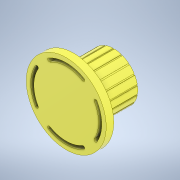
# Autodesk Inventor part: 3inPvcCap
Saved by Autodesk Inventor 2022.2 (Build 262287000, 287)
## iProperties
Created: 2021-11-22
Part Number: 3inPvcCap
Material: PC/ABS Plastic
Document SubType Name: Modeling
Designer: robst
Density: 0.357273 g/cm^3
Appearance: Smooth - Yellow
Author: robst
Autodesk Inventor part; units mm, degrees
ref_plane "YZ Plane" through (0, 0, 0) normal (1, 0, 0) x (0, 1, 0)
ref_plane "XZ Plane" through (0, 0, 0) normal (0, 1, 0) x (-1, 0, 0)
ref_plane "XY Plane" through (0, 0, 0) normal (0, 0, 1) x (1, 0, 0)
sketch "Sketch1" plane through (0, 0, 0) normal (0, 0, 1) x (1, 0, 0)
  circle A0 centre (0, 0) radius 38.1
  circle A1 centre (0, 0) radius 63.5
  circle A2 centre (0, 0) radius 31.75
  dimension "d1" = 76.2
  dimension "d7" = 6.35
  dimension "d45" = 127
  constraints: 3 centre point, 2 coincident
  measures "d1" diameter of A0
  measures "d7" radial gap between concentric circles of A2 A0
  measures "d45" diameter of A1
extrude "Extrusion2" add sketch "Sketch1" along normal blind 12 contours A0 | A1 | A2
extrude "Extrusion3" add sketch "Sketch1" against normal blind 63.5 contours A0
sketch "Sketch6" plane through (0, 0, 12) normal (0, 0, 1) x (1, 0, 0)
  arc A0 (26.9875, 46.7437) -> (-26.9875, 46.7437) centre (0, 0) ccw construction
  arc A1 (28.2638, 48.9544) -> (-28.2639, 48.9544) centre (0, 0) ccw
  arc A2 (25.7111, 44.533) -> (-25.7112, 44.533) centre (0, 0) ccw
  arc A3 (25.7111, 44.533) -> (28.2638, 48.9544) centre (26.9875, 46.7437) ccw
  arc A4 (-28.2639, 48.9544) -> (-25.7112, 44.533) centre (-26.9875, 46.7437) ccw
  line L0 (0, 0) -> (26.9875, 46.7437) construction
  line L1 (0, 0) -> (53.975, 0) construction
  line L2 (0, 0) -> (-26.9875, 46.7437) construction
  dimension "d26" = 53.975
  dimension "d27" = 60
  dimension "d28" = 60
  dimension "d29" = 5.1054
  constraints: 10 point on circle, 6 end point, 5 centre point, 4 tangent, 1 coincident, 1 equal length, 1 horizontal
  measures "d26" radius of A0
  measures "d27" angle of L1 L0
  measures "d28" angle of L0 L2
  measures "d29" diameter of A4
extrude "Extrusion7" cut sketch "Sketch6" against normal through all
pattern_circular "Circular Pattern1" count 4 over 360 about axis through (0, 0, -10) along (0, 0, 1) of "Extrusion7"
sketch "Sketch8" plane through (0, 0, -63.5) normal (0, 0, -1) x (-1, 0, 0)
  circle A0 centre (0, 0) radius 38.1 projected
  arc A1 (0, 38.1) -> (-1.016, 38.0865) centre (0, 0) ccw
  line L0 (0, 0) -> (0, 38.1) construction
  line L1 (0, 38.1) -> (0, 37.084)
  line L2 (0, 37.084) -> (-1.016, 37.084)
  line L3 (-1.016, 37.084) -> (-1.016, 38.0865)
  circle A2 centre (0, 0) radius 38.1 projected
  circle A3 centre (0, 0) radius 38.1
  line L4 (0, 37.084) -> (1.016, 37.084)
  line L5 (1.016, 37.084) -> (1.016, 38.0865)
  dimension "d35" = 1.016
  dimension "d36" = 1.016
  constraints: 12 end point, 3 point on circle, 2 centre point, 2 symmetric about line, 1 coincident, 1 concentric, 1 horizontal, 1 perpendicular, 1 point on line, 1 vertical, 1 other
  measures "d35" distance of L1.end L0.end
  measures "d36" distance of L1.end L2.end
extrude "Extrusion9" cut sketch "Sketch8" against normal up to surface (63.5 mm away) contours L5 L4 L1 A0 | A0 L1 L2 L3
sketch "Sketch3" plane through (0, 0, 12) normal (0, 0, 1) x (1, 0, 0)
  ellipse E0 centre (0, 0) end of major axis (57.15, 0) minor radius 60.8178
  circle A0 centre (0, 0) radius 63.5 projected
  circle A1 centre (0, 0) radius 63.5
  point P0 (-57.15, 0)
  point P1 (57.15, 0)
  dimension "d11" = 60.8178
  dimension "d12" = 57.15
  constraints: 2 coincident, 1 centre point, 1 concentric, 2 other
pattern_circular "Circular Pattern2" count 18 over 360 about axis through (0, 0, -10) along (0, 0, 1) of "Extrusion9"
sketch "Sketch9" plane through (0, 0, 0) normal (0, 0, -1) x (-1, 0, 0)
  point P0 (0, 0)
sketch "Sketch10" plane through (0, 0, 0) normal (0, 0, -1) x (-1, 0, 0)
  circle A0 centre (0, 0) radius 31.75 projected
  arc A1 (-31.497, 4) -> (-31.497, -4) centre (0, 0) ccw
  arc A2 (-4, -31.497) -> (4, -31.497) centre (0, 0) ccw
  arc A3 (31.497, -4) -> (31.497, 4) centre (0, 0) ccw
  arc A4 (4, 31.497) -> (-4, 31.497) centre (0, 0) ccw
  line L0 (-31.497, 4) -> (-4, 4)
  line L1 (4, 4) -> (31.497, 4)
  line L2 (-4, 31.497) -> (-4, 4)
  line L3 (-4, -4) -> (-4, -31.497)
  line L4 (4, 31.497) -> (4, 4)
  line L5 (4, -4) -> (4, -31.497)
  line L6 (-31.497, -4) -> (-4, -4)
  line L7 (4, -4) -> (31.497, -4)
  constraints: 16 end point, 8 point on circle, 4 centre point, 4 parallel, 4 perpendicular, 2 horizontal, 1 coincident, 9 other
extrude "Extrusion10" add sketch "Sketch10" along normal up to surface (63.5 mm away) contours A0 L7 L5 L3 L6 L0 L2 L4 L1
equation "\"d1\" = insideDiameterforPipe"
equation "\"d45\" = outsideDiameter"
equation "\"d8\" = insertDepthIntoPipe"
equation "\"d26\" = slotRadius"
equation "\"d28\" = totalAngleForSlot"
equation "\"d29\" = widthOfSlot"
equation "\"d11\" = 0.5 * elipseMajorDiameter"
equation "\"d12\" = 0.5 * elipseMinorDiameter"
equation "\"insideDiameterforPipe\" = 76.2"
equation "\"outsideDiameter\" = 127"
equation "\"elipseMajorDiameter\" = 121.63552"
equation "\"elipseMinorDiameter\" = 114.3"
equation "\"widthOfSlot\" = 5.1054"
equation "\"totalAngleForSlot\" = 60deg"
equation "\"slotDiameter\" = 0.5 * pipeExteriorDiameter + 0.5 * outsideDiameter"
equation "\"slotRadius\" = 0.5 * slotDiameter"
equation "\"pipeExteriorDiameter\" = 88.9"
equation "\"insertDepthIntoPipe\" = 63.5"
body "Solid2"
